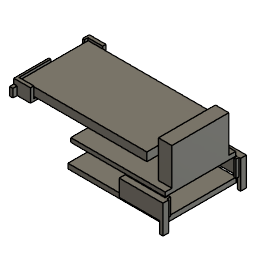
PCB Slot (Autodesk Fusion 360 design; units mm, degrees)
part number: 2026-06-03-15-12-23-460
Autodesk Fusion 360 part; units mm, degrees
note: some values were not read from the file. Chosen so that the rebuilt part matches the saved one: which bodies a step acts on; which face or edge a step refers to.
box "BoxPrimitive1" add length 20 width 37.5 height 2.5 placed x (0, 0, -1) y (-1, 0, 0) z (0, 1, 0) at (-15.1202, 0, 18.4568) makes body 1
box "BoxPrimitive2" add length 21.5 width 28.64 height 2.5 placed x (0, 0, -1) y (-1, 0, 0) z (0, 1, 0) at (-26.36, 0, -25) separate body makes body 2
box "BoxPrimitive3" add length 21 width 28.14 height 2 placed x (0, 0, -1) y (-1, 0, 0) z (0, 1, 0) at (-23.2996, 0, -68.4206) separate body makes body 3
extrude "Extrude6" cut 1 faces at (-32.6796, 2, -75.4206) along direction (0, -1, 0) blind 0.75 on bodies 3 bodies 3
sketch "Sketch5" plane through (0, 1.25, 0) normal (0, 1, 0) x (-1, 0, 0)
  line L0 (23.2996, -89.4206) -> (51.4396, -89.4206)
  line L1 (51.4396, -89.4206) -> (51.4396, -68.4206)
  line L2 (51.4396, -68.4206) -> (23.2996, -68.4206)
  line L3 (23.2996, -68.4206) -> (23.2996, -89.4206)
  line L4 (23.2996, -68.4206) -> (23.2996, -70.4206)
  line L5 (23.2996, -70.4206) -> (27.2996, -70.4206)
  line L6 (27.2996, -70.4206) -> (27.2996, -87.4206)
  line L7 (27.2996, -87.4206) -> (23.2996, -87.4206)
  line L8 (23.2996, -87.4206) -> (23.2996, -70.4206)
  line L9 (51.4396, -89.4206) -> (51.4396, -83.4206)
  line L10 (51.4396, -83.4206) -> (44.4396, -83.4206)
  line L11 (44.4396, -83.4206) -> (44.4396, -74.4206)
  line L12 (44.4396, -74.4206) -> (51.4396, -74.4206)
  line L13 (51.4396, -74.4206) -> (51.4396, -83.4206)
  dimension "d36" = 2
  dimension "d37" = 4
  dimension "d38" = 17
  dimension "d41" = 6
  dimension "d42" = 7
  dimension "d43" = 9
  constraint coincident L2.end L3.start
  constraint perpendicular L2 L4
  constraint horizontal L5
  constraint vertical L6
  constraint horizontal L7
  constraint vertical L8
  constraint coincident L0.end L1.start
  constraint perpendicular L0 L9
  constraint horizontal L10
  constraint vertical L11
  constraint horizontal L12
  constraint vertical L13
  measures "d36" distance of L2.end L4.end
  measures "d37" distance of L4.end L5.end
  measures "d38" distance of L4.end L7.end
  measures "d41" distance of L0.end L9.end
  measures "d42" distance of L9.end L10.end
  measures "d43" distance of L9.end L12.end
extrude "Extrude7" add sketch "Sketch5" along normal blind 11 contours L3 L5 L6 L7 L8 bodies 3
extrude "Extrude8" add sketch "Sketch5" along normal blind 3 contours L1 L10 L11 L12 L13 bodies 3
sketch "Sketch7" plane through (0, 0, 0) normal (0, -1, 0) x (1, 0, 0)
  line L0 (-51.4396, -89.4206) -> (-23.2996, -89.4206)
  line L1 (-23.2996, -89.4206) -> (-23.2996, -68.4206)
  line L2 (-23.2996, -68.4206) -> (-51.4396, -68.4206)
  line L3 (-51.4396, -68.4206) -> (-51.4396, -89.4206)
  line L4 (-51.4396, -89.4206) -> (-51.4396, -84.4206)
  line L5 (-51.4396, -84.4206) -> (-36.4396, -84.4206)
  line L6 (-36.4396, -84.4206) -> (-36.4396, -73.4206)
  line L7 (-36.4396, -73.4206) -> (-51.4396, -73.4206)
  line L8 (-51.4396, -73.4206) -> (-51.4396, -84.4206)
  dimension "d46" = 5
  dimension "d47" = 15
  dimension "d48" = 11
  constraint coincident L0.start L3.end
  constraint perpendicular L0 L4
  constraint horizontal L5
  constraint vertical L6
  constraint horizontal L7
  constraint vertical L8
  measures "d46" distance of L0.start L4.end
  measures "d47" distance of L4.end L5.end
  measures "d48" distance of L4.end L7.end
extrude "Extrude9" add sketch "Sketch7" along normal blind 3 contours L3 L5 L6 L7 L8 bodies 3
extrude "Extrude10" cut 1 faces at (-45.4533, 2.5, -32.1667) along direction (0, -1, 0) blind 1 on bodies 2 bodies 2
move_body "Move1" bodies 2 to x (1, 0, 0) y (0, 1, 0) z (0, 0, 1) at (0, 0, -43.15)
move_body "Move2" bodies 2 to x (1, 0, 0) y (0, 1, 0) z (0, 0, 1) at (3, 0, 0)
move_body "Move3" bodies 2 to x (1, 0, 0) y (0, 1, 0) z (0, 0, 1) at (0, -10, 0)
move_body "Move4" bodies 2 to x (1, 0, 0) y (0, 1, 0) z (0, 0, 1) at (0, 3, 0)
move_body "Move5" bodies 1 to x (1, 0, 0) y (0, 1, 0) z (0, 0, 1) at (-22, 8, -87.25)
move_body "Move6" bodies 1 to x (1, 0, 0) y (0, 1, 0) z (0, 0, 1) at (0, -2, 0)
move_body "Move7" bodies 1 to x (1, 0, 0) y (0, 1, 0) z (0, 0, 1) at (6, 0, 0)
sketch "Sketch9" plane through (0, 0, 0) normal (1, 0, 0) x (0, 0, -1)
  line L0 (68.22, -1, -21) -> (68.22, -2, -21)
  line L1 (68.22, -2, -21) -> (67.95, -2, -21)
  line L2 (67.95, -2, -21) -> (66.45, -2, -21)
  line L3 (66.45, -2, -21) -> (66.45, -1, -21)
  line L4 (66.45, -1, -21) -> (68.22, -1, -21)
  line L5 (89.6213, -1, -21) -> (89.6213, -2, -21)
  line L6 (89.6213, -2, -21) -> (89.85, -2, -21)
  line L7 (89.85, -2, -21) -> (91.35, -2, -21)
  line L8 (91.35, -2, -21) -> (91.35, -1, -21)
  line L9 (91.35, -1, -21) -> (89.6213, -1, -21)
  dimension "d53" = 1
  dimension "d54" = 1.5
  dimension "d55" = 1
  dimension "d56" = 1.5
sketch "Sketch9 (curves -21 mm off its plane)" plane through (-21, 0, 0) normal (1, 0, 0) x (0, 0, -1)
  line L0 (68.22, -1) -> (68.22, -2)
  line L1 (68.22, -2) -> (67.95, -2)
  line L2 (67.95, -2) -> (66.45, -2)
  line L3 (66.45, -2) -> (66.45, -1)
  line L4 (66.45, -1) -> (68.22, -1)
  line L5 (89.6213, -1) -> (89.6213, -2)
  line L6 (89.6213, -2) -> (89.85, -2)
  line L7 (89.85, -2) -> (91.35, -2)
  line L8 (91.35, -2) -> (91.35, -1)
  line L9 (91.35, -1) -> (89.6213, -1)
extrude "Extrude11" add sketch "Sketch9 (curves -21 mm off its plane)" against normal blind 14 separate body makes body 4 at (-25.6667, -2, -90.1975) makes body 5 at (-25.6667, -1, -67.04)
extrude "Extrude12" add 2 faces at (-25.6667, -2, -90.1975) (-25.6667, -2, -67.63) along direction (0, -1, 0) blind 3 on bodies 4 5 bodies 4 5
extrude "Extrude13" add 2 faces at (-25.6667, -1, -90.7738) (-25.6667, -1, -67.04) along direction (0, 1, 0) blind 1 on bodies 4 5 bodies 4 5
extrude "Extrude14" add 2 faces at (-21, -3.3333, -90.1975) (-21, -1.6667, -67.63) along direction (1, 0, 0) blind 1 on bodies 4 5 bodies 4 5
extrude "Extrude15" cut 2 faces at (-20, -3.3333, -90.1975) (-20, -1.6667, -67.63) along direction (-1, 0, 0) blind 1 on bodies 4 5 bodies 4 5
extrude "Extrude16" cut 2 faces at (-21, -3.3333, -90.1975) (-21, -1.6667, -67.63) along direction (-1, 0, 0) blind 2 on bodies 4 5 bodies 4 5
extrude "Extrude17" add 2 faces at (-23, -1.6667, -67.63) (-23, -3.3333, -90.1975) along direction (1, 0, 0) blind 1 on bodies 4 5 bodies 5 4
sketch "Sketch12" plane through (0, -5, 0) normal (0, -1, 0) x (1, 0, 0)
  line L0 (-22, -89.6213) -> (-35, -89.6213)
  line L1 (-35, -89.6213) -> (-35, -91.35)
  line L2 (-35, -91.35) -> (-22, -91.35)
  line L3 (-22, -91.35) -> (-22, -89.6213)
  line L4 (-23, -89.6213) -> (-23, -91.35)
  constraint coincident L0 L4.start
  constraint coincident L2 L4.end
  constraint perpendicular L2 L4
sketch "Sketch13" plane through (0, -5, 0) normal (0, -1, 0) x (1, 0, 0)
  line L0 (-22, -66.45) -> (-35, -66.45)
  line L1 (-35, -66.45) -> (-35, -68.22)
  line L2 (-35, -68.22) -> (-22, -68.22)
  line L3 (-22, -68.22) -> (-22, -66.45)
  line L4 (-23, -68.22) -> (-23, -66.45)
  constraint coincident L2 L4.start
  constraint coincident L0 L4.end
  constraint perpendicular L0 L4
extrude "Extrude18" add sketch "Sketch12" sketch "Sketch13" along normal blind 7 contours L0 L2 L3 L4 of sketch 2 contours L0 L2 L3 L4 bodies 4 5
extrude "Extrude19" cut 1 faces at (-22.3333, -12, -90.1975) along direction (0, 1, 0) blind 4 on bodies 4 bodies 4
extrude "Extrude20" cut 1 faces at (-22.3333, -12, -67.63) along direction (0, 1, 0) blind 4 on bodies 5 bodies 5
extrude "Extrude21" add 2 faces at (-22.3333, -8, -90.1975) (-22.3333, -8, -67.63) along direction (0, -1, 0) blind 0.5 on bodies 4 5 bodies 4 5
sketch "Sketch14" plane through (0, 0, -68.22) normal (0, 0, -1) x (-1, 0, 0)
  line L0 (23, -8.5) -> (23, -5)
  line L1 (23, -5) -> (35, -5)
  line L2 (35, -5) -> (35, 0)
  line L3 (35, 0) -> (22, 0)
  line L4 (22, 0) -> (22, -8.5)
  line L5 (22, -8.5) -> (23, -8.5)
  line L6 (22.5, 0) -> (23.1, 0)
  line L7 (23.1, 0) -> (23.1, -5)
  line L8 (23.1, -5) -> (22.5, -5)
  line L9 (22.5, -5) -> (22.5, 0)
  constraint horizontal L6
  constraint vertical L7
  constraint horizontal L8
  constraint vertical L9
  constraint coincident L1 L7.end
  constraint coincident L3 L6.start
extrude "Extrude22" add sketch "Sketch14" along normal blind 21.5 contours L1 L3 L6 L7 L8 L9 bodies 4 5
extrude "Extrude23" cut sketch "Sketch14" along normal blind 20.5 contours L1 L3 L6 L7 L8 L9 bodies 4 makes body 6 at (-26.6667, -1.6667, -68.22)
extrude "Extrude24" add sketch "Sketch14" along normal blind 1 contours L1 L3 L6 L7 L8 L9 bodies 6
move_body "Move8" bodies 1 to x (1, 0, 0) y (0, 1, 0) z (0, 0, 1) at (-9, 0, 0)
move_body "Move9" bodies 1 to x (1, 0, 0) y (0, 1, 0) z (0, 0, 1) at (6, 0, 0)
sketch "Sketch15" plane through (0, 0, 0) normal (0, 0, 1) x (1, 0, 0)
  line L0 (-72.5, 9, -90) -> (-67.5, 9, -90)
  line L1 (-67.5, 9, -90) -> (-67.5, 5, -90)
  line L2 (-67.5, 5, -90) -> (-72.5, 5, -90)
  line L3 (-72.5, 5, -90) -> (-72.5, 9, -90)
  line L4 (-71.9, 9, -90) -> (-71.9, 5, -90)
  line L5 (-72.5, 5.7, -90) -> (-67.5, 5.7, -90)
sketch "Sketch15 (curves -90 mm off its plane)" plane through (0, 0, -90) normal (0, 0, 1) x (1, 0, 0)
  line L0 (-72.5, 9) -> (-67.5, 9)
  line L1 (-67.5, 9) -> (-67.5, 5)
  line L2 (-67.5, 5) -> (-72.5, 5)
  line L3 (-72.5, 5) -> (-72.5, 9)
  line L4 (-71.9, 9) -> (-71.9, 5)
  line L5 (-72.5, 5.7) -> (-67.5, 5.7)
extrude "Extrude25" add sketch "Sketch15 (curves -90 mm off its plane)" along normal blind 1 separate body makes body 7
extrude "Extrude26" add sketch "Sketch15 (curves -90 mm off its plane)" against normal blind 2 contours L0 L3 L4 L5 | L2 L3 L4 L5 | L1 L2 L4 L5 bodies 7
move_body "Move10" bodies 7 to x (1, 0, 0) y (0, 1, 0) z (0, 0, 1) at (0, 0, -1)
extrude "Extrude27" add 1 faces at (-70.6333, 5.2333, -93) along direction (0, 0, -1) blind 0.5 on bodies 7 bodies 7
extrude "Extrude28" add 1 faces at (-70.6333, 5.2333, -93.5) along direction (0, 0, -1) blind 5 on bodies 7 bodies 7
extrude "Extrude29" add 1 faces at (-70.6333, 5.2333, -98.5) along direction (0, 0, -1) blind 2 on bodies 7 bodies 7
move_body "Move11" bodies 7 to x (1, 0, 0) y (0, 1, 0) z (0, 0, 1) at (0, 0, 16)
move_body "Move12" bodies 7 to x (1, 0, 0) y (0, 1, 0) z (0, 0, 1) at (0, 0, 6)
move_body "Move13" bodies 7 to x (1, 0, 0) y (0, 1, 0) z (0, 0, 1) at (0, 0, 0.5)
extrude "Extrude30" add sketch "Sketch15 (curves -90 mm off its plane)" against normal blind 1 separate body makes body 8
extrude "Extrude31" add sketch "Sketch15 (curves -90 mm off its plane)" along normal blind 0.5 contours L0 L3 L4 L5 | L2 L3 L4 L5 | L1 L2 L4 L5 bodies 8
extrude "Extrude32" add 1 faces at (-70.6333, 5.2333, -89.5) along direction (0, 0, 1) blind 0.5 on bodies 8 bodies 8
move_body "Move14" bodies 8 to x (1, 0, 0) y (0, 1, 0) z (0, 0, 1) at (0, 0, 0.8)
move_body "Move15" bodies 8 to x (1, 0, 0) y (0, 1, 0) z (0, 0, 1) at (0, 0, 0.2)
sketch "Sketch16" plane through (0, 0, -90) normal (0, 0, -1) x (-1, 0, 0)
  line L0 (67.5, 5) -> (72.5, 5)
  line L1 (72.5, 5) -> (72.5, 9)
  line L2 (72.5, 9) -> (67.5, 9)
  line L3 (67.5, 9) -> (67.5, 5)
  line L4 (72.5, 5) -> (71.5, 5)
  line L5 (71.5, 5) -> (71.5, 7.5)
  line L6 (71.5, 7.5) -> (72.5, 7.5)
  line L7 (72.5, 7.5) -> (72.5, 5)
  constraint horizontal L4
  constraint vertical L5
  constraint horizontal L6
  constraint vertical L7
  constraint coincident L0.end L1.start
extrude "Extrude33" add sketch "Sketch16" along normal blind 1.25 contours L0 L1 L4 L5 L6 L7 bodies 8
sketch "Sketch17" plane through (0, 0, -67.5) normal (0, 0, 1) x (1, 0, 0)
  line L0 (-72.5, 5) -> (-67.5, 5)
  line L1 (-67.5, 5) -> (-67.5, 9)
  line L2 (-67.5, 9) -> (-72.5, 9)
  line L3 (-72.5, 9) -> (-72.5, 5)
  line L4 (-72.5, 5) -> (-71.5, 5)
  line L5 (-71.5, 5) -> (-71.5, 7.5)
  line L6 (-71.5, 7.5) -> (-72.5, 7.5)
  line L7 (-72.5, 7.5) -> (-72.5, 5)
  dimension "d103" = 1
  dimension "d104" = 2.5
  constraint horizontal L4
  constraint vertical L5
  constraint horizontal L6
  constraint vertical L7
  constraint coincident L0.start L3.end
  measures "d103" distance of L0.start L4.end
  measures "d104" distance of L0.start L6.end
extrude "Extrude34" add sketch "Sketch17" along normal blind 1.25 contours L0 L3 L4 L5 L6 L7 bodies 7
move_body "Move16" bodies 1 to x (1, 0, 0) y (0, 1, 0) z (0, 0, 1) at (5, 0, 0)
move_body "Move17" bodies 8 7 to x (1, 0, 0) y (0, 1, 0) z (0, 0, 1) at (5, 0, 0)
